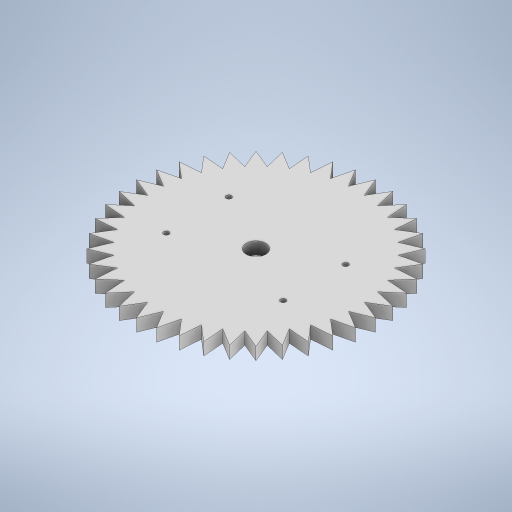
# Autodesk Inventor part: BIG ASS GEAR
Saved by Autodesk Inventor 2023 (Build 270158030, 158C)
## iProperties
Created: 2022-10-06
Part Number: BIG ASS GEAR
Material: Generic
Document SubType Name: Modeling
Designer: cjj5381
Density: 1 g/cm^3
Appearance: Default
Author: cjj5381
Autodesk Inventor part; units mm, degrees
ref_plane "YZ Plane" through (0, 0, 0) normal (1, 0, 0) x (0, 1, 0)
ref_plane "XZ Plane" through (0, 0, 0) normal (0, 1, 0) x (-1, 0, 0)
ref_plane "XY Plane" through (0, 0, 0) normal (0, 0, 1) x (1, 0, 0)
sketch "Sketch1" plane through (0, 0, 0) normal (0, 1, 0) x (-1, 0, 0)
  circle A0 centre (0, 0) radius 101.6
  dimension "d0" = 203.2
  constraints: 1 centre point, 1 coincident
  measures "d0" diameter of A0
extrude "Extrusion1" add sketch "Sketch1" along normal blind 12.7
sketch "Sketch2" plane through (0, 12.7, 0) normal (0, 1, 0) x (1, 0, 0)
  line L0 (-8.4294, 101.2497) -> (0, 121.6)
  line L1 (0, 121.6) -> (8.4294, 101.2497)
  circle A0 centre (0, 0) radius 101.6 projected
  line L2 (0, 0) -> (0, 122.8461)
  circle A1 centre (0, 0) radius 101.6 projected
  arc A2 (8.4294, 101.2497) -> (-8.4294, 101.2497) centre (0, 0) ccw
  point P0 (0, 101.6)
  dimension "d3" = 45
  dimension "d4" = 20
  constraints: 6 end point, 4 point on circle, 1 centre point, 1 concentric, 1 point on line, 1 symmetric about line, 1 vertical, 2 other
  measures "d3" angle of L0 L1
  measures "d4" distance of L0.end point (0, 101.6)
extrude "Extrusion2" add sketch "Sketch2" against normal up to surface (12.7 mm away) contours L0 L2 A0 | L1 A0 L2
pattern_circular "Circular Pattern1" count 40 over 360 about axis through (0, 0, 0) along (0, 1, 0) of "Extrusion2"
sketch "Sketch3" plane through (0, 12.7, 0) normal (0, 1, 0) x (1, 0, 0)
  circle A0 centre (0, 0) radius 10
  dimension "d10" = 20
  constraints: 1 centre point, 1 coincident
  measures "d10" diameter of A0
extrude "Extrusion3" cut sketch "Sketch3" against normal through all
sketch "Sketch5" plane through (0, 12.7, 0) normal (0, 1, 0) x (1, 0, 0)
  line L0 (-59.436, 31.75) -> (59.436, 31.75)
  line L1 (59.436, 31.75) -> (59.436, -31.75)
  line L2 (59.436, -31.75) -> (-59.436, -31.75)
  line L3 (-59.436, -31.75) -> (-59.436, 31.75)
  circle A0 centre (0, 0) radius 10 projected
  line L4 (-59.436, 31.75) -> (59.436, -31.75) construction
  line L5 (59.436, 31.75) -> (-59.436, -31.75) construction
  dimension "d22" = 63.5
  dimension "d23" = 118.872
  constraints: 12 end point, 4 coincident, 2 midpoint, 2 parallel, 1 horizontal, 1 perpendicular
  measures "d22" distance of L0.end L1.end
  measures "d23" distance of L1.end L2.end
hole "Hole1" at (-59.436, 12.7, -31.75) at (-59.436, 12.7, 31.75) at (59.436, 12.7, 31.75) at (59.436, 12.7, -31.75) direction (0, -1, 0) diameter 5.5 end through all clearance for "Countersunk Flat Head Screw ISO 2009/7046" size "M5" standard "ISO"
body "Solid1"
